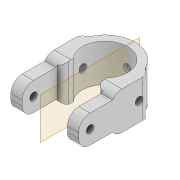
# Autodesk Inventor part: Arm_clip
Saved by Autodesk Inventor 2022 (Build 260153000, 153)
## iProperties
Created: 2022-07-25
Part Number: Arm_clip
Material: Generic
Document SubType Name: Modeling
Designer: dell
Density: 1 g/cm^3
Appearance: Default
Mass: 0.914716 g
Surface Area: 10.3779 cm^2
Volume: 0.914716 cm^3
Author: dell
Autodesk Inventor part; units mm, degrees
ref_plane "XZ Plane" through (0, 0, 0) normal (0, 1, 0) x (-1, 0, 0)
ref_plane "XY Plane" through (0, 0, 0) normal (0, 0, 1) x (1, 0, 0)
sketch "Sketch1" plane through (0, 0, 0) normal (0, 1, 0) x (-1, 0, 0)
  circle A0 centre (0, 0) radius 6
  circle A1 centre (0, 0) radius 8
  line L0 (8, 0) -> (-8, 0)
  line L1 (-8, 0) -> (-8, 16)
  line L2 (-8, 16) -> (8, 16)
  line L3 (8, 16) -> (8, 0)
  line L4 (6, 0) -> (-6, 0)
  line L5 (-6, 0) -> (-6, 16)
  line L6 (-6, 16) -> (6, 16)
  line L7 (6, 16) -> (6, 0)
  line L8 (4.5, 3.9686) -> (4.5, 6.6144)
  line L9 (-4.5, 3.9686) -> (-4.5, 6.6144)
  line L10 (4.5, 6.6144) -> (6, 6.6144)
  line L11 (-4.5, 6.6144) -> (-6, 6.6144)
  line L12 (-11.2, 0) -> (11.2, 0) projected
  dimension "d0" = 12
  dimension "d1" = 2
  dimension "d3" = 8
  dimension "d4" = 1.5
  dimension "d5" = 1.5
  constraints: 24 end point, 8 point on circle, 6 point on line, 5 parallel, 3 perpendicular, 2 centre point, 1 coincident, 1 collinear, 1 horizontal, 1 vertical
  measures "d0" diameter of A0
  measures "d1" radial gap between concentric circles of A0 A1
  measures "d3" distance edge to line of A1 L2
  measures "d4" distance between parallel lines of L7 L8
  measures "d5" distance between parallel lines of L5 L9
extrude "Extrusion1" add sketch "Sketch1" along normal blind 10 contours L0 A1 A0 | L7 A1 L0 | A0 L8 A1 L7 | L5 A1 L9 A0 | L0 A1 L5 | A1 L7 L2 L3 | A1 L10 L7 | L1 L2 L5 A1 | L5 L11 A1
fillet "Fillet1" radius 1.5 2 edges at (-4.5, 5, 6.6144) (4.5, 5, 6.6144)
sketch "Sketch2" plane through (6, 0, 16) normal (-1, 0, 0) x (0, 0, 1)
  line L0 (0, 0) -> (0, 10) projected
  circle A0 centre (-3, 5) radius 1
  line L1 (-9.3856, 0) -> (-9.3856, 10) projected
  line L2 (-9.3856, 0) -> (0, 0) projected
  line L3 (-9.3856, 10) -> (0, 10) projected
  point P0 (-16, 0)
  dimension "d9" = 2
  dimension "d10" = 2
  dimension "d28" = 5
  constraints: 1 centre point
  measures "d9" diameter of A0
  measures "d10" distance edge to line of A0 L0
  measures "d28" distance from line of L2 A0.centre
extrude "Extrusion2" cut sketch "Sketch2" along normal mid plane 100 contours A0
sketch "Sketch4" plane through (-8, 0, 0) normal (-1, 0, 0) x (0, 0, 1)
  circle A0 centre (13, 5) radius 1 projected
  line L0 (0, 0) -> (16, 0) projected
  line L1 (16, 0) -> (16, 10) projected
  line L2 (0, 10) -> (16, 10) projected
  line L3 (0, 0) -> (0, 10) projected
  line L4 (0, 0) -> (0, 0) projected
  line L5 (0, 0) -> (0, 10) projected
  line L6 (0, 10) -> (0, 10) projected
  line L7 (0, 0) -> (0, 10) projected
  line L8 (0, 0) -> (0, 10) projected
  line L9 (0, 10) -> (0, 0)
  line L10 (0, 0) -> (-3, 0)
  line L11 (-3, 0) -> (-3, 10)
  line L12 (-3, 10) -> (0, 10)
  point P0 (0, 0)
  dimension "d22" = 3
  constraints: 8 end point, 3 equal length, 1 perpendicular
  measures "d22" distance between parallel lines of L5 L11
extrude "Extrusion3" add sketch "Sketch4" along normal mid plane 2
fillet "Fillet2" radius 2 2 edges at (-9, 5, -3) (-7.4162, 5, -3)
mirror "Mirror1" about plane through (0, 0, 0) normal (1, 0, 0) of "Extrusion3", "Fillet2"
sketch "Sketch7" plane through (0, 0, 0) normal (1, 0, 0) x (0, 1, 0)
  circle A0 centre (5, 0) radius 1
  line L0 (-2, 0) -> (12, 0) projected
  point P0 (0, 0)
  dimension "d30" = 2
  dimension "d31" = 5
  constraints: 1 centre point, 1 midpoint
  measures "d30" diameter of A0
  measures "d31" distance of point (0, 0) A0.centre
extrude "Extrusion6" cut sketch "Sketch7" along normal mid plane 100
sketch "Sketch8" plane through (0, 10, 0) normal (0, 1, 0) x (1, 0, 0)
  line L0 (-6, -16) -> (-6, -6.6144) projected
  line L1 (-9, 1.0438) -> (-9, -16) projected
  line L2 (-6, -16) -> (-9, -16)
  line L3 (-9, -16) -> (-9, -7)
  line L4 (-9, -7) -> (-6, -7)
  line L5 (-6, -7) -> (-6, -16)
  line L6 (9, -16) -> (9, 1.0438) projected
  line L7 (6, -16) -> (9, -16)
  line L8 (9, -16) -> (9, -7)
  line L9 (9, -7) -> (6, -7)
  line L10 (6, -7) -> (6, -16)
  point P0 (0, 0)
  dimension "d34" = 9
  dimension "d35" = 9
  constraints: 16 end point, 4 parallel, 2 horizontal, 2 perpendicular, 2 point on line
  measures "d34" distance between parallel lines of L2 L4
  measures "d35" distance between parallel lines of L7 L9
extrude "Extrusion7" cut sketch "Sketch8" against normal blind 1.3
sketch "Sketch9" plane through (0, 0, 0) normal (0, -1, 0) x (1, 0, 0)
  line L0 (6, 16) -> (9, 16) projected
  line L1 (9, -1.0438) -> (9, 16) projected
  line L2 (6, 16) -> (9, 16)
  line L3 (9, 16) -> (9, 7)
  line L4 (9, 7) -> (6, 7)
  line L5 (6, 7) -> (6, 16)
  line L6 (-6, 16) -> (-6, 6.6144) projected
  line L7 (-9, -1.0438) -> (-9, 16) projected
  line L8 (-6, 16) -> (-9, 16)
  line L9 (-9, 16) -> (-9, 7)
  line L10 (-9, 7) -> (-6, 7)
  line L11 (-6, 7) -> (-6, 16)
  point P0 (0, 0)
  dimension "d38" = 9
  dimension "d39" = 9
  constraints: 16 end point, 4 parallel, 2 horizontal, 2 perpendicular, 2 point on line
  measures "d38" distance between parallel lines of L0 L4
  measures "d39" distance between parallel lines of L8 L10
extrude "Extrusion8" cut sketch "Sketch9" against normal blind 1.3
fillet "Fillet5" radius 3 8 edges at (7.5, 8.7, 16) (7.5, 1.3, 16) (-7.5, 8.7, 16) (-7.5, 1.3, 16) (7.5, 0, 7) (7.5, 10, 7) (-7.5, 10, 7) (-7.5, 0, 7)
sketch "Sketch10" plane through (0, 0, 0) normal (0, 0, 1) x (1, 0, 0)
  circle A0 centre (0, 5) radius 1
  point P0 (0, 0)
  dimension "d42" = 2
  dimension "d43" = 5
  constraints: 1 centre point
  measures "d42" diameter of A0
  measures "d43" distance of point (0, 0) A0.centre
extrude "Extrusion9" cut sketch "Sketch10" against normal blind 100
body "Solid1"
